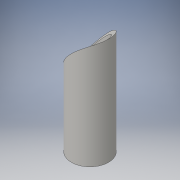
# Autodesk Inventor part: Angled Pipe (Attached to Control Pipe)
Saved by Autodesk Inventor 2016 (Build 200138000, 138)
## iProperties
Created: 2017-09-28
Part Number: Angled Pipe (Attached to Control Pipe)
Material: Generic
Document SubType Name: Modeling
Designer: Student
Density: 1 g/cm^3
Appearance: Default
Author: Student
Autodesk Inventor part; units mm, degrees
ref_plane "XZ Plane" through (0, 0, 0) normal (0, 1, 0) x (-1, 0, 0)
ref_plane "XY Plane" through (0, 0, 0) normal (0, 0, 1) x (1, 0, 0)
sketch "Sketch1" plane through (0, 0, 0) normal (0, 1, 0) x (-1, 0, 0)
  circle A0 centre (0, 0) radius 20.066
  circle A1 centre (0, 0) radius 24.2951
  dimension "d0" = 40.132
  dimension "d1" = 48.5902
  constraints: 2 centre point, 2 coincident
  measures "d0" diameter of A0
  measures "d1" diameter of A1
extrude "Extrusion1" add sketch "Sketch1" along normal blind 152.4
ref_plane "Work Plane4" through (15.0868, 167.4868, 0) normal (0.7071068, 0.7071068, 0) x (0, 0, -1)
ref_plane "Work Plane3" through (0, 152.4, 0) normal (0.7071068, 0.7071068, 0) x (0, 0, -1)
sketch "Sketch2" plane through (15.0868, 167.4868, 0) normal (0.7071068, 0.7071068, 0) x (0, 0, -1)
  ellipse E0 centre (0, 0) end of major axis (24.2951, 0) minor radius 17.1792 projected
  line L0 (0, -17.1792) -> (46.559, -17.1792)
  line L1 (0, -17.1792) -> (-63.5901, -17.1792)
  line L2 (0, -17.1792) -> (0, 39.92)
  line L3 (0, 39.92) -> (57.0992, 39.92)
  arc A0 (-57.0992, 39.92) -> (57.0992, 39.92) centre (0, 39.92) ccw
  line L4 (57.0992, 39.92) -> (-57.0992, 39.92)
  point P0 (0, -107.7631)
  dimension "d6" = 57.0992
  dimension "d7" = 57.0992
  dimension "d8" = 114.1984
  constraints: 10 end point, 6 horizontal, 3 point on circle, 1 centre point, 1 point on line, 1 vertical, 1 vertical alignment, 1 other
  measures "d6" distance of L0.start L2.end
  measures "d7" distance of L2.end L3.end
  measures "d8" distance of L3.end L4.end
extrude "Extrusion2" cut sketch "Sketch2" against normal blind 152.4
sketch "Sketch3" plane through (0, 0, 0) normal (0, -1, 0) x (1, 0, 0)
  circle A0 centre (0, 0) radius 77.6216
  constraints: 1 centre point, 1 coincident
extrude "Extrusion3" cut sketch "Sketch3" against normal blind 63.5
sketch "Sketch4" plane through (0, 63.5, 0) normal (0, -1, 0) x (1, 0, 0)
  circle A0 centre (0, 0) radius 20.066
  circle A1 centre (0, 0) radius 24.2951
  constraints: 2 centre point, 2 coincident
extrude "Extrusion4" add sketch "Sketch4" along normal blind 50.8
ref_plane "Work Plane1" through (0, 76.2, 0) normal (0, 1, 0) x (1, 0, 0)
ref_plane "Work Plane2" through (0, 152.4, 0) normal (0, 1, 0) x (1, 0, 0)
body "Solid1"
